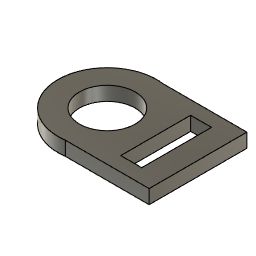
Excersise 1 v1 (Autodesk Fusion 360 design; units mm, degrees)
Autodesk Fusion 360 part; units mm, degrees
sketch "Sketch1" plane through (0, 0, 0) normal (0, 0, 1) x (1, 0, 0)
  line L0 (0, 0) -> (-60, 0)
  line L1 (-60, 0) -> (-60, 70)
  line L2 (-60, 70) -> (0, 70)
  line L3 (0, 70) -> (0, 0)
  arc A0 (-60, 70) -> (-60, 0) centre (-64.9382, 35) ccw
  circle A1 centre (-64.9382, 35) radius 19.958
  line L4 (-30.6239, 60.2944) -> (-15.6239, 60.2944)
  line L5 (-15.6239, 60.2944) -> (-15.6239, 10.2944)
  line L6 (-15.6239, 10.2944) -> (-30.6239, 10.2944)
  line L7 (-30.6239, 10.2944) -> (-30.6239, 60.2944)
  dimension "d1" = 70
  dimension "d2" = 60
  dimension "d3" = 50
  dimension "d4" = 15
  constraint horizontal L0
  constraint vertical L1
  constraint horizontal L2
  constraint vertical L3
  constraint coincident L0.start L3.end
  constraint concentric A0 A1
  constraint horizontal L4
  constraint vertical L5
  constraint horizontal L6
  constraint vertical L7
  measures "d1" distance of L0.start L2.end
  measures "d2" distance of L0.start L0.end
  measures "d3" distance of L4.start L6.end
  measures "d4" distance of L4.start L4.end
sketch "Sketch2" plane through (0, 0, 0) normal (0, 0, 1) x (1, 0, 0)
extrude "Extrude1" add sketch "Sketch1" along normal blind 10 contours L0 L1 L2 L3 A1 | L1 A0 A1
